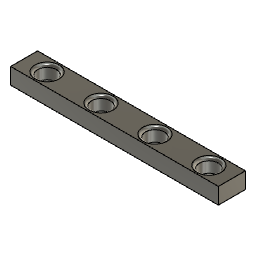
LEDx4 v1 (Autodesk Fusion 360 design; units mm, degrees)
Autodesk Fusion 360 part; units mm, degrees
note: some values were not read from the file. Set by a fixed rule: which face or edge a step refers to.
sketch "Sketch1" plane through (0, 0, 0) normal (0, 0, 1) x (1, 0, 0)
  line L0 (0.4954, 7.8418) -> (38.9954, 7.8418)
  line L1 (38.9954, 7.8418) -> (38.9954, 12.8418)
  line L2 (38.9954, 12.8418) -> (0.4954, 12.8418)
  line L3 (0.4954, 12.8418) -> (0.4954, 7.8418)
  line L4 (19.7454, 12.8418) -> (19.7454, 7.8418) construction
  line L5 (0.4954, 10.3418) -> (38.9954, 10.3418) construction
  line L6 (19.7454, 10.3418) -> (0.4954, 10.3418) construction
  circle A0 centre (10.1204, 10.3418) radius 1.5
  circle A1 centre (19.7454, 10.3418) radius 1.5
  line L7 (19.7454, 10.3418) -> (38.9954, 10.3418) construction
  circle A2 centre (29.3704, 10.3418) radius 1.5 construction
  circle A3 centre (29.3704, 10.3418) radius 1.75
  dimension "d1" = 38.5
  dimension "d2" = 5
  dimension "d3" = 3
  dimension "d4" = 3
  dimension "d5" = 3
  constraint horizontal L0
  constraint vertical L1
  constraint horizontal L2
  constraint vertical L3
  constraint midpoint L2 L4.start
  constraint midpoint L0 L4.end
  constraint midpoint L3 L5.start
  constraint midpoint L1 L5.end
  constraint midpoint L4 L6.start
  constraint midpoint L6 A0.centre
  constraint coincident L6.start A1.centre
  constraint midpoint L7 A2.centre
  constraint concentric A2 A3
  measures "d1" distance of L0.start L0.end
  measures "d2" distance of L0.start L2.end
  measures "d3" diameter of A0
  measures "d4" diameter of A1
  measures "d5" diameter of A2
extrude "Extrude1" add sketch "Sketch1" along normal blind 3
fillet "Fillet1" radius 0.5 3 faces at (31.1182, 10.2545, 2) (21.2435, 10.267, 2) (11.6185, 10.267, 2)
move_face "OffsetFaces1" offset -0.25 1 faces at (11.6129, 10.1924, 1.1667)
move_face "OffsetFaces2" offset -0.25 1 faces at (21.2379, 10.1924, 1.1667)
delete_face "DeleteFace1" 2 faces at (31.4623, 9.5804, 2.9994) (12.2777, 9.7924, 2.9994)
extrude "Extrude2" add 1 faces at (0.4954, 9.5084, 2) along direction (1, 0, 0) blind 15
extrude "Extrude3" add 1 faces at (38.9954, 9.5084, 1) along direction (-1, 0, 0) blind 14.5
sketch "Sketch2" plane through (0, 0, 3) normal (0, 0, 1) x (-1, 0, 0)
  line L0 (-38.9954, -12.8418) -> (-0.4954, -12.8418)
  line L1 (-0.4954, -12.8418) -> (-0.4954, -7.8418)
  line L2 (-0.4954, -7.8418) -> (-38.9954, -7.8418)
  line L3 (-38.9954, -7.8418) -> (-38.9954, -12.8418)
  circle A0 centre (-19.7454, -10.3418) radius 2.25
  line L4 (-19.7454, -10.3418) -> (-4.7454, -10.3418) construction
  line L5 (-4.7454, -10.3418) -> (-34.7454, -10.3418) construction
  circle A1 centre (-34.7454, -10.3418) radius 1.75
  circle A2 centre (-4.7454, -10.3418) radius 1.75
  dimension "d16" = 15
  dimension "d17" = 30
  dimension "d18" = 3.5
  dimension "d19" = 3.5
  constraint coincident A0.centre L4.start
  constraint parallel L0 L4
  constraint parallel L4 L5
  constraint coincident L5.end A1.centre
  constraint coincident L4.end L5.start
  measures "d16" distance of A0.centre L4.end
  measures "d17" distance of L4.end L5.end
  measures "d18" diameter of A1
  measures "d19" diameter of A2
extrude "Extrude4" cut sketch "Sketch2" against normal blind 8 contours A1 | A2
fillet "Fillet2" radius 0.5 2 edges at (6.3769, 9.7089, 3) (36.3769, 9.7089, 3)
fillet "Fillet3" radius 0.5 2 edges at (36.3769, 10.9746, 0) (6.3769, 10.9746, 0)
extrude "Extrude5" add 1 faces at (38.9954, 9.5084, 1) along direction (-1, 0, 0) blind 23
sketch "Sketch3" plane through (0, 0, 3) normal (0, 0, 1) x (-1, 0, 0)
  line L0 (-38.9954, -12.8418) -> (-0.4954, -12.8418)
  line L1 (-0.4954, -12.8418) -> (-0.4954, -7.8418)
  line L2 (-0.4954, -7.8418) -> (-38.9954, -7.8418)
  line L3 (-38.9954, -7.8418) -> (-38.9954, -12.8418)
  circle A0 centre (-4.7454, -10.3418) radius 2.25
  line L4 (-4.7454, -10.3418) -> (-34.7454, -10.3418) construction
  line L5 (-4.7454, -10.3418) -> (-19.7454, -10.3418) construction
  line L6 (-4.7454, -10.3418) -> (-12.2454, -10.3418) construction
  line L7 (-4.7454, -10.3418) -> (-14.7454, -10.3418) construction
  line L8 (-34.7454, -10.3418) -> (-24.7454, -10.3418) construction
  circle A1 centre (-14.7454, -10.3418) radius 1.75
  circle A2 centre (-24.7454, -10.3418) radius 1.75
  circle A3 centre (-34.7454, -10.3418) radius 1.75
  dimension "d28" = 30
  dimension "d29" = 15
  dimension "d30" = 7.5
  dimension "d31" = 10
  dimension "d32" = 10
  dimension "d33" = 3.5
  dimension "d34" = 3.5
  dimension "d35" = 3.5
  constraint coincident A0.centre L4.start
  constraint parallel L0 L4
  constraint parallel L4 L5
  constraint parallel L5 L6
  constraint parallel L4 L7
  constraint perpendicular L3 L8
  constraint coincident L7.end A1.centre
  constraint coincident L8.end A2.centre
  constraint coincident L4.end L8.start
  measures "d28" distance of A0.centre L4.end
  measures "d29" distance of A0.centre L5.end
  measures "d30" distance of A0.centre L6.end
  measures "d31" distance of A0.centre L7.end
  measures "d32" distance of L4.end L8.end
  measures "d33" diameter of A1
  measures "d34" diameter of A2
  measures "d35" diameter of A3
extrude "Extrude6" cut sketch "Sketch3" against normal blind 10 contours A1 | A2 | A3
fillet "Fillet4" radius 0.5 3 edges at (16.3769, 9.7089, 3) (26.3769, 9.7089, 3) (36.3769, 9.7089, 3)
fillet "Fillet5" radius 0.5 3 edges at (36.3769, 10.9746, 0) (26.3769, 10.9746, 0) (16.3769, 10.9746, 0)
